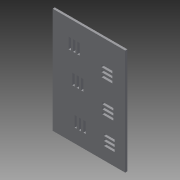
# Autodesk Inventor part: Top
Saved by Autodesk Inventor 2015 (Build 190159000, 159)
## iProperties
Created: 2014-09-15
Part Number: Top
Material: Generic
Document SubType Name: Modeling
Designer: ehagerup
Density: 1 g/cm^3
Appearance: Default
Author: ehagerup
Autodesk Inventor part; units mm, degrees
ref_plane "YZ Plane" through (0, 0, 0) normal (1, 0, 0) x (0, 1, 0)
ref_plane "XZ Plane" through (0, 0, 0) normal (0, 1, 0) x (-1, 0, 0)
ref_plane "XY Plane" through (0, 0, 0) normal (0, 0, 1) x (1, 0, 0)
sketch "Sketch1" plane through (0, 0, 0) normal (0, 1, 0) x (-1, 0, 0)
  line L0 (55.4221, -22.8509) -> (55.4221, -25.3509)
  line L1 (-7.557, 11.8403) -> (92.5214, 11.8403)
  line L2 (92.5214, 11.8403) -> (92.5214, -134.0855)
  line L3 (92.5214, -134.0855) -> (-7.557, -134.0855)
  line L4 (-7.557, -134.0855) -> (-7.557, 11.8403)
  line L5 (24.9643, -21.3009) -> (9.9643, -21.3009)
  line L6 (9.9643, -21.3009) -> (9.9643, -24.3009)
  line L7 (9.9643, -24.3009) -> (24.9643, -24.3009)
  line L8 (24.9643, -24.3009) -> (24.9643, -21.3009)
  line L9 (24.9643, -27.3009) -> (9.9643, -27.3009)
  line L10 (9.9643, -27.3009) -> (9.9643, -30.3009)
  line L11 (9.9643, -30.3009) -> (24.9643, -30.3009)
  line L12 (24.9643, -30.3009) -> (24.9643, -27.3009)
  line L13 (9.9643, -36.3009) -> (24.9643, -36.3009)
  line L14 (24.9643, -36.3009) -> (24.9643, -33.3009)
  line L15 (24.9643, -33.3009) -> (9.9643, -33.3009)
  line L16 (9.9643, -33.3009) -> (9.9643, -36.3009)
  line L17 (23.8002, -65.0745) -> (8.8002, -65.0745)
  line L18 (8.8002, -65.0745) -> (8.8002, -68.0745)
  line L19 (8.8002, -68.0745) -> (23.8002, -68.0745)
  line L20 (23.8002, -68.0745) -> (23.8002, -65.0745)
  line L21 (8.8002, -71.0745) -> (23.8002, -71.0745)
  line L22 (23.8002, -71.0745) -> (23.8002, -74.0745)
  line L23 (23.8002, -74.0745) -> (8.8002, -74.0745)
  line L24 (8.8002, -74.0745) -> (8.8002, -71.0745)
  line L25 (23.8002, -77.0745) -> (8.8002, -77.0745)
  line L26 (8.8002, -77.0745) -> (8.8002, -80.0745)
  line L27 (8.8002, -80.0745) -> (23.8002, -80.0745)
  line L28 (23.8002, -80.0745) -> (23.8002, -77.0745)
  line L29 (21.7165, -101.8292) -> (6.7165, -101.8292)
  line L30 (6.7165, -101.8292) -> (6.7165, -104.8292)
  line L31 (6.7165, -104.8292) -> (21.7165, -104.8292)
  line L32 (21.7165, -104.8292) -> (21.7165, -101.8292)
  line L33 (6.7165, -107.8292) -> (21.7165, -107.8292)
  line L34 (21.7165, -107.8292) -> (21.7165, -110.8292)
  line L35 (21.7165, -110.8292) -> (6.7165, -110.8292)
  line L36 (6.7165, -110.8292) -> (6.7165, -107.8292)
  line L37 (21.7165, -113.8292) -> (6.7165, -113.8292)
  line L38 (6.7165, -113.8292) -> (6.7165, -116.8292)
  line L39 (6.7165, -116.8292) -> (21.7165, -116.8292)
  line L40 (21.7165, -116.8292) -> (21.7165, -113.8292)
  line L41 (64.4221, -10.6009) -> (61.4221, -10.6009)
  line L42 (61.4221, -10.6009) -> (61.4221, -25.6009)
  line L43 (61.4221, -25.6009) -> (64.4221, -25.6009)
  line L44 (64.4221, -25.6009) -> (64.4221, -10.6009)
  line L45 (55.4221, -10.6009) -> (58.4221, -10.6009)
  line L46 (58.4221, -10.6009) -> (58.4221, -25.6009)
  line L47 (58.4221, -25.6009) -> (55.4221, -25.6009)
  line L48 (55.4221, -25.6009) -> (55.4221, -10.6009)
  line L49 (70.4221, -10.6009) -> (67.4221, -10.6009)
  line L50 (67.4221, -10.6009) -> (67.4221, -25.6009)
  line L51 (67.4221, -25.6009) -> (70.4221, -25.6009)
  line L52 (70.4221, -25.6009) -> (70.4221, -10.6009)
  line L53 (50.3229, -51.1341) -> (53.3229, -51.1341)
  line L54 (53.3229, -51.1341) -> (53.3229, -66.1341)
  line L55 (53.3229, -66.1341) -> (50.3229, -66.1341)
  line L56 (50.3229, -66.1341) -> (50.3229, -51.1341)
  line L57 (59.3229, -51.1341) -> (56.3229, -51.1341)
  line L58 (56.3229, -51.1341) -> (56.3229, -66.1341)
  line L59 (56.3229, -66.1341) -> (59.3229, -66.1341)
  line L60 (59.3229, -66.1341) -> (59.3229, -51.1341)
  line L61 (65.3229, -51.1341) -> (62.3229, -51.1341)
  line L62 (62.3229, -51.1341) -> (62.3229, -66.1341)
  line L63 (62.3229, -66.1341) -> (65.3229, -66.1341)
  line L64 (65.3229, -66.1341) -> (65.3229, -51.1341)
  line L65 (62.1773, -100.1635) -> (59.1773, -100.1635)
  line L66 (59.1773, -100.1635) -> (59.1773, -115.1635)
  line L67 (59.1773, -115.1635) -> (62.1773, -115.1635)
  line L68 (62.1773, -115.1635) -> (62.1773, -100.1635)
  line L69 (56.1773, -100.1635) -> (53.1773, -100.1635)
  line L70 (53.1773, -100.1635) -> (53.1773, -115.1635)
  line L71 (53.1773, -115.1635) -> (56.1773, -115.1635)
  line L72 (56.1773, -115.1635) -> (56.1773, -100.1635)
  line L73 (47.1773, -115.1635) -> (50.1773, -115.1635)
  line L74 (50.1773, -115.1635) -> (50.1773, -100.1635)
  line L75 (50.1773, -100.1635) -> (47.1773, -100.1635)
  line L76 (47.1773, -100.1635) -> (47.1773, -115.1635)
  point P0 (0, 0)
  constraints: 154 end point, 38 parallel, 19 horizontal, 19 perpendicular
extrude "Extrusion1" add sketch "Sketch1" along normal blind 3
body "Solid1"
